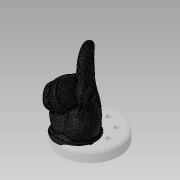
# Autodesk Inventor part: Pointing_Finger
Saved by Autodesk Inventor 2017 (Build 210142000, 142)
## iProperties
Part Number: Pointing_Finger
Material: Generisch
Document SubType Name: Modeling
Designer: Max
Density: 1 g/cm^3
Appearance: Vorgabe
Author: Max
Autodesk Inventor part; units mm, degrees
ref_plane "YZ Plane" through (0, 0, 0) normal (1, 0, 0) x (0, 1, 0)
ref_plane "XZ Plane" through (0, 0, 0) normal (0, 1, 0) x (-1, 0, 0)
ref_plane "XY Plane" through (0, 0, 0) normal (0, 0, 1) x (1, 0, 0)
sketch "Skizze1" plane through (-4.3917, 11.7982, 0) normal (0, 0, -1) x (-1, 0, 0)
  circle A0 centre (-0.2488, -4.8451) radius 16.9829
  point P0 (-4.3917, -11.7982)
  constraints: 1 centre point, 1 coincident
extrude "Extrusion1" add sketch "Skizze1" along normal blind 4 and the other way blind 2
fillet "Rundung1" radius 2 1 edges at (12.8401, 6.9531, 2)
sketch "Skizze2" plane through (-4.1429, 6.9531, 2) normal (0, 0, 1) x (1, 0, 0)
  circle A0 centre (0, 0) radius 14.9829 construction
  point P0 (4.1429, -6.9531)
  point P1 (0, 11)
  dimension "d5" = 11
  measures "d5" distance of A0.centre point (0, 11)
hole "Bohrung1" at (-4.1429, 17.9531, 2) direction (0, 0, -1) diameter 2.9 end through all clearance for "Inbusschraube ISO 4762" size "M2.5" standard "ISO"
pattern_circular "Runde Anordnung1" count 8 over 360 about axis through (-4.1429, 6.9531, 0) along (0, 0, -1) of "Bohrung1"
